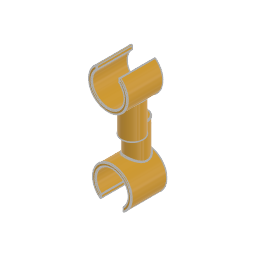
LEGO Minifigure (Autodesk Fusion 360 archive; units mm, degrees)
design "Lesson 16"
part number: 2026-03-11-20-05-45-624
part number: 2026-03-11-20-06-27-128
Autodesk Fusion 360 part; units mm, degrees
note: some values were not read from the file. Set by a fixed rule: which sketch regions a step uses.
sketch "Sketch1" plane through (0, 0, 0) normal (0, 1, 0) x (1, 0, 0) in component "Left HAND"
  circle A0 centre (0, 0) radius 1.7272
  circle A1 centre (0, 0) radius 1.397
  line L0 (-0.9525, -1.4408) -> (-0.9525, -1.0219)
  line L1 (0, 0) -> (0, -1.524) construction
  line L2 (0.9525, -1.4408) -> (0.9525, -1.0219)
  dimension "d1" = 3.4544
  dimension "d2" = 2.794
  dimension "d3" = 1.905
  constraint coincident A0.centre A1.centre
  constraint coincident A0 L0.start
  constraint coincident A1 L0.end
  constraint vertical L0
  constraint vertical L1
  constraint symmetric L0.start L1 L2.start
  constraint symmetric L0.end L1 L2.end
  measures "d1" diameter of A0
  measures "d2" diameter of A1
  measures "d3" distance of L0 L2
extrude "Extrude1" add sketch "Sketch1" along normal blind 1.016 and the other way blind 2.159 contours A0 A1 L0 L2 picked at (-1.1455, -1.1363) makes body 1 in component "Left HAND"
sketch "Sketch2" plane through (0, 0, 0) normal (0, 0, 1) x (1, 0, 0) in component "Left HAND"
  circle A0 centre (0, 0) radius 0.9525
  dimension "d8" = 1.905
  constraint coincident A0.centre origin
  measures "d8" diameter of A0
extrude "Extrude2" add sketch "Sketch2" against normal blind 4.445 bodies 1 in component "Left HAND"
delete_face "DeleteFace1" 1 faces at (-0.0029, 0.9525, -0.4657) on bodies 1 in component "Left HAND"
fillet "Fillet1" radius 0.0635 2 edges at (-0.888, 0.3444, -4.445) (0.9525, 0, -1.4408) 4 faces at (0, -2.159, -1.6141) (-0.9525, -0.0423, 1.1616) (0.9525, -1.1007, 1.3012) (0, 1.016, -1.6141) on bodies 1 in component "Left HAND"
mirror "MirrorComponent1" about plane through (0, 0, 0) normal (0, 0, 1) of bodies 1 makes body 2 in component "Right HAND"
component "Left HAND" placed x (1, 0, 0) y (0, 1, 0) z (0, 0, 1) at (0, 0, 0)
component "Right HAND" placed x (1, 0, 0) y (0, 1, 0) z (0, 0, 1) at (0, 0, -8.89)
equation "d1 = ( 0.068 * 2 ) * 1 in"
equation "d2 = ( 0.055 * 2 ) * 1 in"

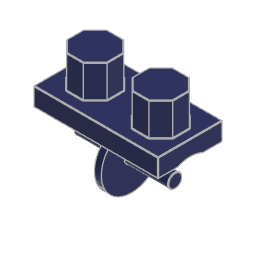
design "Lesson 13"
part number: 2026-03-11-18-58-51-171
Autodesk Fusion 360 part; units mm, degrees
sketch "Sketch1" plane through (0, 0, 0) normal (0, 0, 1) x (1, 0, 0)
  line L0 (7.239, -3.7465) -> (-7.239, -3.7465)
  line L1 (-7.239, -3.7465) -> (-7.239, 3.7465)
  line L2 (-7.239, 3.7465) -> (7.239, 3.7465)
  line L3 (7.239, 3.7465) -> (7.239, -3.7465)
  line L4 (7.239, -3.7465) -> (-7.239, 3.7465) construction
  line L5 (-7.239, -3.7465) -> (7.239, 3.7465) construction
  dimension "d1" = 14.478
  dimension "d2" = 7.493
  constraint horizontal L0
  constraint perpendicular L0 L1
  constraint parallel L0 L2
  constraint parallel L1 L3
  constraint coincident L4 origin
  constraint coincident L5 origin
  measures "d1" distance of L1.end L2.end
  measures "d2" distance of L0.end L1.end
extrude "Extrude1" add sketch "Sketch1" against normal blind 2.159
sketch "Sketch2" plane through (0, 0, 0) normal (0, 0, 1) x (-1, 0, 0)
  line L0 (-7.239, -3.7465) -> (7.239, -3.7465)
  line L1 (7.239, -3.7465) -> (7.239, 3.7465)
  line L2 (7.239, 3.7465) -> (-7.239, 3.7465)
  line L3 (-7.239, 3.7465) -> (-7.239, -3.7465)
  circle A0 centre (-3.81, 0) radius 2.54 construction
  line L4 (-6.1567, 0.972) -> (-6.1567, -0.972)
  line L5 (-6.1567, -0.972) -> (-4.782, -2.3467)
  line L6 (-4.782, -2.3467) -> (-2.838, -2.3467)
  line L7 (-2.838, -2.3467) -> (-1.4633, -0.972)
  line L8 (-1.4633, -0.972) -> (-1.4633, 0.972)
  line L9 (-1.4633, 0.972) -> (-2.838, 2.3467)
  line L10 (-2.838, 2.3467) -> (-4.782, 2.3467)
  line L11 (-4.782, 2.3467) -> (-6.1567, 0.972)
  line L12 (0, -2.5) -> (0, -20)
  line L13 (4.782, -2.3467) -> (2.838, -2.3467)
  line L14 (2.838, -2.3467) -> (1.4633, -0.972)
  line L15 (1.4633, -0.972) -> (1.4633, 0.972)
  line L16 (1.4633, 0.972) -> (2.838, 2.3467)
  line L17 (2.838, 2.3467) -> (4.782, 2.3467)
  line L18 (4.782, 2.3467) -> (6.1567, 0.972)
  line L19 (6.1567, 0.972) -> (6.1567, -0.972)
  line L20 (6.1567, -0.972) -> (4.782, -2.3467)
  point P0 (-3.81, 0)
  dimension "d5" = 5.08
  dimension "d6" = 3.81
  constraint coincident P0 A0.centre
  constraint coincident A0 L4.start
  constraint horizontal L10
  constraint horizontal origin A0.centre
  constraint symmetric L4.start L12 L18.end
  constraint symmetric L4.end L12 L19.end
  constraint symmetric L5.end L12 L13.start
  constraint symmetric L6.end L12 L13.end
  constraint symmetric L7.end L12 L14.end
  constraint symmetric L8.end L12 L15.end
  constraint symmetric L9.end L12 L16.end
  constraint symmetric L10.end L12 L17.end
  measures "d5" diameter of A0
  measures "d6" distance of origin A0.centre
extrude "Extrude2" add sketch "Sketch2" along normal blind 3.81 contours L4 L5 L6 L7 L8 L9 L10 L11 | L13 L14 L15 L16 L17 L18 L19 L20
sketch "Sketch3" plane through (0, 0, 0) normal (1, 0, 0) x (0, 1, 0)
  circle A0 centre (0, -5.334) radius 3.5052
  line L0 (3.7465, 0) -> (-3.7465, 0)
  dimension "d9" = 7.0104
  dimension "d10" = 5.334
  constraint vertical origin A0.centre
  measures "d9" diameter of A0
  measures "d10" distance of A0.centre L0
extrude "Extrude3" cut sketch "Sketch3" along normal through all and the other way through all
extrude "Extrude4" add sketch "Sketch3" along normal mid plane 0.8128
sketch "Sketch4" plane through (0.4064, 0, 0) normal (1, 0, 0) x (0, 1, 0)
  arc A0 (-1.4852, -2.159) -> (1.4852, -2.159) centre (0, -5.334) ccw
  arc A1 (1.4852, -2.159) -> (-1.4852, -2.159) centre (0, -5.334) ccw
  circle A2 centre (0, -5.08) radius 0.8255
  dimension "d14" = 1.651
  measures "d14" diameter of A2
extrude "Extrude5" add sketch "Sketch4" along normal blind 5.08 contours A2
mirror "Mirror1" about plane through (0, 0, 0) normal (1, 0, 0) of "Extrude5"
fillet "Fillet1" radius 0.0635 2 edges at (-5.4864, -0.7696, -5.3785) (5.4864, -0.7696, -5.3785) 7 faces at (-3.0278, -0.324, 3.81) (3.0278, 0.324, 3.81) (2.413, -3.7465, -0.7197) (7.239, 0, -0.6096) (-2.413, 3.7465, -0.7197) (-7.239, 0, -0.6096) (-0.946, -3.2799, 0)

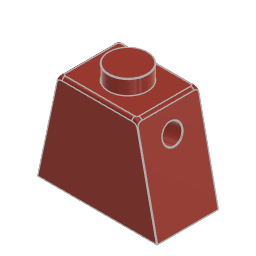
design "Lesson 12"
part number: 2026-03-11-18-38-59-440
Autodesk Fusion 360 part; units mm, degrees
sketch "Sketch1" plane through (0, 0, 0) normal (0, 1, 0) x (1, 0, 0)
  line L0 (0, 0) -> (0, -12.7)
  line L1 (-5.08, -12.7) -> (5.08, -12.7)
  line L2 (-7.7795, 0) -> (7.7795, 0)
  line L3 (-5.08, -12.7) -> (-7.7795, 0)
  line L4 (5.08, -12.7) -> (7.7795, 0)
  dimension "d1" = 12.7
  dimension "d2" = 10.16
  dimension "d3" = 78
  dimension "d4" = 78
  constraint coincident L0.start origin
  constraint vertical L0
  constraint perpendicular L0 L1
  constraint coincident L0.end L1
  constraint perpendicular L0 L2
  constraint coincident L0.start L2
  constraint symmetric L0 L2.start L2.end
  measures "d1" distance of L0.start L0.end
  measures "d2" distance of L1.start L1.end
  measures "d3" angle of L2 L4
  measures "d4" angle of L2 L3
extrude "Extrude1" add sketch "Sketch1" along normal mid plane 8.001
sketch "Sketch2" plane through (0, 0, 12.7) normal (0, 0, 1) x (-1, 0, 0)
  line L0 (-5.08, 4.0005) -> (-5.08, -4.0005)
  line L1 (-5.08, -4.0005) -> (5.08, -4.0005)
  line L2 (5.08, -4.0005) -> (5.08, 4.0005)
  line L3 (5.08, 4.0005) -> (-5.08, 4.0005)
  circle A0 centre (0, 0) radius 2.54
  dimension "d7" = 5.08
  constraint coincident A0.centre origin
  measures "d7" diameter of A0
extrude "Extrude2" add sketch "Sketch2" along normal blind 1.905 contours A0
sketch "Sketch3" plane through (0, 0, 0) normal (0, 0, -1) x (1, 0, 0)
  line L0 (-7.7795, 4.0005) -> (-7.7795, -4.0005)
  line L1 (-7.7795, -4.0005) -> (7.7795, -4.0005)
  line L2 (7.7795, -4.0005) -> (7.7795, 4.0005)
  line L3 (7.7795, 4.0005) -> (-7.7795, 4.0005)
  circle A0 centre (-3.81, 0) radius 2.54
  circle A1 centre (3.81, 0) radius 2.54
  dimension "d10" = 5.08
  dimension "d11" = 5.08
  dimension "d12" = 3.81
  dimension "d13" = 3.81
  constraint horizontal origin A0.centre
  constraint horizontal origin A1.centre
  measures "d10" diameter of A0
  measures "d11" diameter of A1
  measures "d12" distance of origin A1.centre
  measures "d13" distance of origin A0.centre
extrude "Extrude3" cut sketch "Sketch3" against normal blind 5.08 contours A0 | A1
sketch "Sketch5" plane through (0, -4.0005, 0) normal (0, -1, 0) x (1, 0, 0)
  line L0 (5.08, 12.7) -> (-5.08, 12.7)
  line L1 (-5.08, 12.7) -> (-7.7795, 0)
  line L2 (-7.7795, 0) -> (7.7795, 0)
  line L3 (7.7795, 0) -> (5.08, 12.7)
  line L4 (0, 0) -> (0, 0.6409)
  line L5 (-0.0557, 0) -> (-0.0557, 9.525)
  line L6 (-0.0557, 9.525) -> (5.7549, 9.525) construction
  dimension "d16" = 9.525
  constraint coincident L4.start origin
  constraint perpendicular L2 L4
  constraint coincident L2 L5.start
  constraint perpendicular L2 L5
  constraint coincident L3 L6.end
  constraint perpendicular L5 L6
  measures "d16" distance of L5.start L5.end
sketch "Sketch6" plane through (7.4432, 0, 1.5821) normal (0.978148, 0, 0.207912) x (0, 1, 0)
  line L0 (-4.0005, -1.6174) -> (4.0005, -1.6174)
  line L1 (4.0005, -1.6174) -> (4.0005, 11.3663)
  line L2 (4.0005, 11.3663) -> (-4.0005, 11.3663)
  line L3 (-4.0005, 11.3663) -> (-4.0005, -1.6174)
  line L4 (-4.0005, 8.1084) -> (0, 8.1084)
  constraint coincident L3 L4.start
  constraint perpendicular L3 L4
  constraint vertical origin L4.end
hole "Hole1" at (5.7573, 0, 9.5133) direction (-0.978148, 0, -0.207912) diameter 2.54 depth 5.08 tip angle 180
mirror "Mirror1" about plane through (0, 0, 0) normal (1, 0, 0) of "Hole1"
fillet "Fillet1" radius 0.381 4 edges at (0, 4.0005, 12.7) (-5.08, 0, 12.7) (0, -4.0005, 12.7) (5.08, 0, 12.7)
fillet "Fillet1" radius 0.0635 7 edges at (-6.4297, 4.0005, 6.35) (-6.4297, -4.0005, 6.35) (6.4297, 4.0005, 6.35) (6.4297, -4.0005, 6.35) (5.6619, -1.1841, 9.9626) (-5.8528, -1.1841, 9.0641) (2.3681, 0.9185, 14.605) 1 faces at (1.0816, 3.4924, 0)
equation "d10 = d11"
equation "d13 = d12"
equation "d18 = ( 0.05 * 2 ) * 1 in"

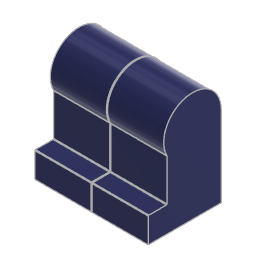
design "Lesson 14"
part number: 2026-03-11-19-15-29-438
part number: 2026-03-11-19-17-35-052
Autodesk Fusion 360 part; units mm, degrees
sketch "Sketch1" plane through (0, 0, 0) normal (1, 0, 0) x (0, 1, 0) in component "Left  LEG"
  line L0 (3.5052, 0.8672) -> (3.5052, -9.9278)
  line L1 (3.5052, -9.9278) -> (-5.3848, -9.9278)
  line L2 (-5.3848, -9.9278) -> (-5.3848, -6.7528)
  line L3 (-5.3848, -6.7528) -> (-3.0988, -6.7528)
  line L4 (-3.0988, -6.7528) -> (-3.0988, -1.6383)
  arc A0 (3.5052, 0) -> (-3.0988, -1.6383) centre (0, 0) ccw
  dimension "d1" = 7.0104
  dimension "d2" = 10.795
  dimension "d3" = 8.89
  dimension "d4" = 3.175
  dimension "d5" = 6.604
  constraint coincident A0.centre origin
  constraint vertical L0
  constraint tangent L0 A0
  constraint perpendicular L0 L1
  constraint perpendicular L1 L2
  constraint perpendicular L2 L3
  constraint perpendicular L3 L4
  constraint coincident L0 A0.start
  measures "d1" diameter of A0
  measures "d2" distance of L0.start L0.end
  measures "d3" distance of L0.end L1.end
  measures "d4" distance of L1.end L2.end
  measures "d5" distance of L0 L4
extrude "Extrude1" add sketch "Sketch1" along normal blind 6.9088 makes body 1 in component "Left  LEG"
sketch "Sketch2" plane through (0, 0, 0) normal (-1, 0, 0) x (0, -1, 0) in component "Left  LEG"
  line L0 (-3.5052, 0) -> (-3.5052, -9.9278)
  line L1 (-3.5052, -9.9278) -> (5.3848, -9.9278)
  line L2 (5.3848, -9.9278) -> (5.3848, -6.7528)
  line L3 (5.3848, -6.7528) -> (3.0988, -6.7528)
  line L4 (3.0988, -6.7528) -> (3.0988, -1.6383)
  arc A0 (3.0988, -1.6383) -> (-3.5052, 0) centre (0, 0) ccw
  circle A1 centre (0, 0) radius 0.8255
  dimension "d8" = 1.651
  constraint concentric A0 A1
  measures "d8" diameter of A1
extrude "Extrude2" cut sketch "Sketch2" against normal blind 5.08 contours A1 bodies 1 in component "Left  LEG"
fillet "Fillet1" radius 0.0635 4 edges at (0, -0.844, 3.4021) (0, 3.5052, -4.9639) (3.4544, -3.0988, -6.7528) (3.4544, -5.3848, -6.7528) 2 faces at (0, 0.1967, -5.8285) (4.6059, 0.5419, -9.9278) on bodies 1 in component "Left  LEG"
mirror "MirrorComponent1" about plane through (0, 0, 0) normal (0, 0, 1) of bodies 1 makes body 2 in component "Right LEG"
component "Left  LEG" placed x (1, 0, 0) y (0, 1, 0) z (0, 0, 1) at (0, 0, 0)
component "Right LEG" placed x (-1, 0, 0) y (0, 1, 0) z (0, 0, -1) at (0, 0, 0)
equation "d1 = 0.138 * 2 in"
